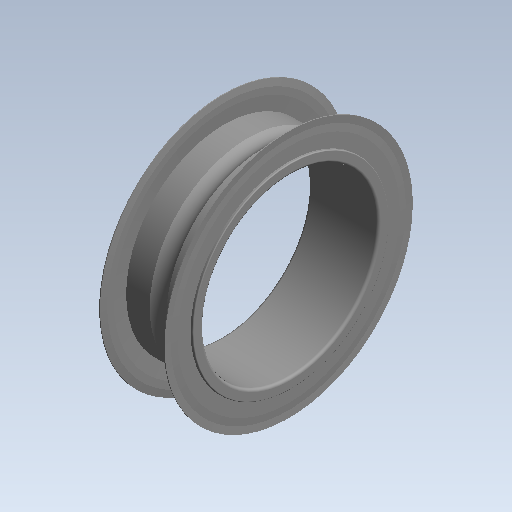
# Autodesk Inventor part: W 61700 X-2RS1_PART1
Saved by Autodesk Inventor 2021 (Build 250183000, 183)
## iProperties
Part Number: W 61700 X-2RS1_PART1
Material: Allgemein
Catalog Web Link: www.cadenas.de
Description: -Deep groove ball bearings
Vendor: SKF
Document SubType Name: Modeling
Designer: partserver
Manufacturer: SKF
Mass: 0.084907 g
Surface Area: 5.42965 cm^2
Volume: 0.084907 cm^3
Density: 1 g/cm^3
Appearance: PSOLRGB-175-175-175
Category: PARTsolutions
Company: SKF
PSOL_IDENT_0: {$CADENAS_DATA\23d-libs\skf_r32\bearings_units_and_housings\ball_bearings\deep_groove_ball_bearings\
PSOL_IDENT_1: bb1_001_101.prj},207 {VTYP=3D},{NB=W 61700 X-2RS1_PART1},{LINA=W 61700 X-2RS1_PART1},{NN=BB1_001_101
PSOL_IDENT_2: _PART1},{NOPRJ=TRUE},{DATE=12.05.2020 07:47:22},{GEOMDATE=07.04.2020 07:08:50},{VERSION=},{LINEID=18
PSOL_IDENT_3: 530},{WBVAR=},{WBNUMERIC=}  {NB=W 61700 X-2RS1_PART1},{LINA=W 61700 X-2RS1_PART1},{KT=DUMMY},{DESIGN
PSOL_IDENT_4: ATION=W 61700 X-2RS1},{DD=10.000},{D=15.000},{B=4.000},{C=0.000},{DD1=11.21},{DD2=0.00},{D1=0.00},{D
PSOL_IDENT_5: 2=14.20},{D3=0.000},{D4=0.000},{HH=MIN},{BB=0.000},{FF=0.00},{R0MAX=MIN},{R0=MIN},{R12=0.15},{PITCH=
PSOL_IDENT_6: 12.49},{DW=1.588},{DDAMIN=11.000},{DDAMAX=11.000},{DDBMIN=MIN},{DDBMAX=MIN},{DBMIN=MIN},{DAMAX=14.50
PSOL_IDENT_7: 0},{BBAMIN=MIN},{CAMAX=MIN},{RAMAX=0.150},{LOAD1=0.488},{LOAD2=0.220},{LOAD3=0.009},{SPEED1=MIN},{SP
PSOL_IDENT_8: EED2=24000},{KR=0.015},{F0=8.000},{Z=11},{II=1},{MASS=0.002},{BEARING=W 61700 X-2RS1},{RING=},{HELP=
PSOL_IDENT_9: 0.723},{HELP2=0.400},{DD1ALG=5.605},{YALG=5.605},{PITCH1=12.490},{DW1=1.588},{YALG1=6.777},{HALG1=0.
PSOL_IDENT_10: 723},{SH=5.605},{CU=0.482},{DESIGN=dgbbw2rs},{HALG=0.605},{B1=0},{SHIELDHELP=2}
NB: W 61700 X-2RS1_PART1
NT: Deep groove ball bearings
NBSYN: $DESIGNATION._PART1
LINA: W 61700 X-2RS1_PART1
CATALOG: SKF
SUPPLIER: SKF
ARTICLENO: W 61700 X-2RS1_PART1
BOMINFO: W 61700 X-2RS1_PART1
CREATOR: CADENAS GmbH
Title: W 61700 X-2RS1_PART1
Author: Cadenas PARTsolutions
Comments: Deep groove ball bearings
Autodesk Inventor part; units mm, degrees
ref_plane "YZ Plane" through (0, 0, 0) normal (1, 0, 0) x (0, 1, 0)
ref_plane "XZ Plane" through (0, 0, 0) normal (0, 1, 0) x (-1, 0, 0)
ref_plane "XY Plane" through (0, 0, 0) normal (0, 0, 1) x (1, 0, 0)
sketch "Sketch_12" plane through (0, 0, 0) normal (0, 0, 1) x (1, 0, 0)
  line L0 (50, 0) -> (-50, 0)
  line L1 (0, 5.555) -> (0, 5.15)
  arc A0 (0, 5.15) -> (0.15, 5) centre (0.15, 5.15) ccw
  line L2 (0.15, 5) -> (3.85, 5)
  arc A1 (3.85, 5) -> (4, 5.15) centre (3.85, 5.15) ccw
  line L3 (4, 5.15) -> (4, 5.555)
  arc A2 (4, 5.555) -> (3.95, 5.605) centre (3.95, 5.555) ccw
  line L4 (3.95, 5.605) -> (2.4699, 5.605)
  arc A3 (1.5301, 5.605) -> (2.4699, 5.605) centre (2, 6.245) ccw
  line L5 (1.5301, 5.605) -> (0.05, 5.605)
  arc A4 (0.05, 5.605) -> (0, 5.555) centre (0.05, 5.555) ccw
  constraints: 12 end point, 10 point on circle, 5 centre point
revolve "Revolution1" add sketch "Sketch_12" angle 360 about axis through (50, 0, 0) along (1, 0, 0)
sketch "Sketch_15" plane through (0, 0, 0) normal (0, 0, 1) x (1, 0, 0)
  line L0 (50, 0) -> (-50, 0)
  line L1 (0.135, 7.1) -> (0.1575, 6.7263)
  line L2 (0.1575, 6.7263) -> (0.135, 6.3525)
  line L3 (0.135, 6.3525) -> (0.135, 5.605)
  line L4 (0.135, 5.605) -> (0.18, 5.605)
  line L5 (0.18, 5.605) -> (0.225, 6.3525)
  line L6 (0.225, 6.3525) -> (0.225, 6.7263)
  line L7 (0.225, 6.7263) -> (0.18, 7.1)
  line L8 (0.18, 7.1) -> (0.135, 7.1)
  constraints: 18 end point
revolve "Revolution2" add sketch "Sketch_15" angle 360 about axis through (50, 0, 0) along (1, 0, 0)
sketch "Sketch_16" plane through (0, 0, 0) normal (0, 0, 1) x (1, 0, 0)
  line L0 (50, 0) -> (-50, 0)
  line L1 (3.775, 6.7263) -> (3.775, 6.3525)
  line L2 (3.775, 6.3525) -> (3.82, 5.605)
  line L3 (3.82, 5.605) -> (3.865, 5.605)
  line L4 (3.865, 5.605) -> (3.865, 6.3525)
  line L5 (3.865, 6.3525) -> (3.8425, 6.7263)
  line L6 (3.8425, 6.7263) -> (3.865, 7.1)
  line L7 (3.865, 7.1) -> (3.82, 7.1)
  line L8 (3.82, 7.1) -> (3.775, 6.7263)
  constraints: 18 end point
revolve "Revolution3" add sketch "Sketch_16" angle 360 about axis through (50, 0, 0) along (1, 0, 0)
body "Solid1"
